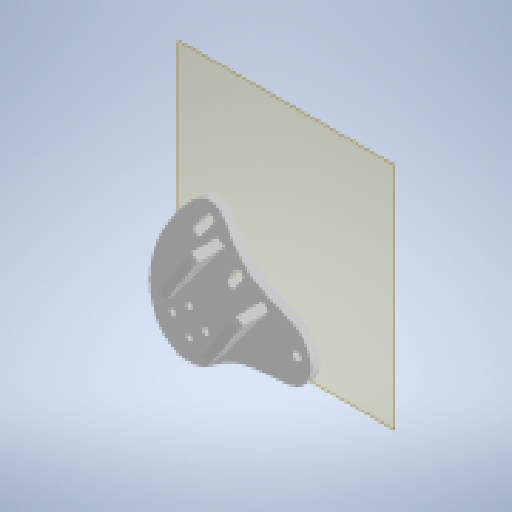
# Autodesk Inventor part: Soporte motor 2
Saved by Autodesk Inventor 2025.3 (Build 293356000, 356)
## iProperties
Created: 2025-11-13
Part Number: Soporte motor 2
Material: Generic
Document SubType Name: Modeling
Designer: juanm
Density: 1 g/cm^3
Appearance: Default
Author: juanm
Autodesk Inventor part; units mm, degrees
ref_plane "YZ Plane" through (0, 0, 0) normal (1, 0, 0) x (0, 1, 0)
ref_plane "XZ Plane" through (0, 0, 0) normal (0, 1, 0) x (-1, 0, 0)
ref_plane "XY Plane" through (0, 0, 0) normal (0, 0, 1) x (1, 0, 0)
ref_plane "Work Plane1" through (0, 0, 0) normal (0, 0, 1) x (1, 0, 0)
sketch "Sketch1" plane through (0, 0, 0) normal (0, 0, 1) x (1, 0, 0)
  circle A0 centre (-25.0838, -31.7051) radius 2.5 projected
  circle A1 centre (-43.012, -13.2629) radius 2.5 projected
  circle A2 centre (-44.8914, 13.7567) radius 2.5 projected
  circle A3 centre (-28.0838, 36.7109) radius 2.5 projected
  circle A4 centre (0.8935, 43.7288) radius 2.5 projected
  circle A5 centre (29.5533, 30.4373) radius 2.5 projected
  circle A6 centre (43.6662, -0.0951) radius 2.5 projected
  circle A7 centre (47.6662, -52.5951) radius 2.5 projected
  circle A8 centre (10.6662, -52.5951) radius 2.5 projected
  circle A9 centre (-6.8338, -0.0951) radius 8.75 projected
  line L0 (56.6662, -60.0951) -> (51.1662, -0.0951) projected
  spline S0 degree 4 poles (51.1662, -0.0951) (50.0319, 24.6801) (26.25, 55.8136) (-25.1104, 60.0951) (-56.6662, 18.5311) (-54.7055, -22.2338) (-29.645, -43.1708) (-8.3823, -44.3792) (3.1662, -40.8213) knots 0 0 0 0 0 0.330099 0.457579 0.582312 0.704438 0.895347 0.895347 0.895347 0.895347 0.895347 projected
  line L1 (3.1662, -40.8213) -> (3.1662, -60.0951) projected
  line L2 (3.1662, -60.0951) -> (56.6662, -60.0951) projected
  circle A10 centre (-6.8338, -0.0951) radius 80 construction
  circle A11 centre (-51.3856, -66.5416) radius 20
  spline S1 degree 4 poles (-67.6748, -78.146) (-80.1343, -60.6563) (-73.4442, -28.8039) (-34.6199, 23.5084) (-28.149, -22.306) (-1.1527, -34.0954) (21.6131, -40.077) (20.0804, -79.4594) (-16.1771, -65.3424) (-30.503, -75.865) (-39.3686, -82.5289) knots 0 0 0 0 0 0.227581 0.363335 0.480166 0.59047 0.703016 0.817261 1 1 1 1 1
  line L3 (10.6662, -52.5951) -> (-43.012, -13.2629) construction
  line L4 (-25.0838, -31.7051) -> (10.6662, -52.5951) construction
  line L5 (10.6662, -52.5951) -> (-42.0733, -6.3735) construction
  line L6 (10.6662, -52.5951) -> (-49.6403, -16.0265) construction
  arc A12 (-37.4996, -10.382) -> (-40.9954, -14.7405) centre (10.6662, -52.5951) ccw
  arc A13 (-40.9954, -14.7405) -> (-44.098, -19.3872) centre (10.6662, -52.5951) ccw
  arc A14 (-41.2598, -7.0865) -> (-45.0286, -11.7853) centre (10.6662, -52.5951) ccw
  arc A15 (-45.0286, -11.7853) -> (-48.3734, -16.7947) centre (10.6662, -52.5951) ccw
  arc A16 (-37.4996, -10.382) -> (-41.2598, -7.0865) centre (-39.3797, -8.7342) ccw
  arc A17 (-48.3734, -16.7947) -> (-44.098, -19.3872) centre (-46.2357, -18.0909) ccw
  line L7 (10.6662, -52.5951) -> (-30.2455, -33.2568) construction
  line L8 (10.6662, -52.5951) -> (-26.0132, -26.6253) construction
  arc A18 (-21.0867, -30.1134) -> (-24.5082, -35.9687) centre (10.6662, -52.5951) ccw
  arc A19 (-25.1674, -27.2241) -> (-29.0287, -33.832) centre (10.6662, -52.5951) ccw
  arc A20 (-21.0867, -30.1134) -> (-25.1674, -27.2241) centre (-23.1271, -28.6687) ccw
  arc A21 (-29.0287, -33.832) -> (-24.5082, -35.9687) centre (-26.7685, -34.9004) ccw
  point P0 (0, 0)
  point P1 (-60.5912, -17.8314)
  point P2 (-36.7792, -0.096)
  point P3 (-23.1279, -18.1974)
  point P4 (0.0342, -33.7731)
  point P5 (16.7837, -45.8922)
  point P6 (15.1081, -64.5601)
  point P7 (-10.6842, -70.5676)
  point P8 (-45.0286, -11.7853)
  point P9 (-21.0867, -30.1134)
  dimension "d0" = 160
  dimension "d1" = 40
  dimension "d2" = 5
  dimension "d3" = 5
  dimension "d4" = 2.5
  dimension "d5" = 5
  dimension "d6" = 5
  constraints: 27 point on circle, 15 point on line, 12 end point, 11 centre point, 7 coincident, 4 tangent, 13 other
  measures "d1" diameter of A11
  measures "d2" angle of L5 L3
  measures "d3" angle of L6 L3
  measures "d4" radius of A16
  measures "d5" angle of L4 L7
  measures "d6" angle of L4 L8
extrude "Extrusion1" add sketch "Sketch1" along normal blind 5 contours A15 A17 S0 S1 L2 L1 A13 A12 A16 A14 | A11 | A17 S0 L1 L2 S1 A11
sketch "Sketch2" plane through (0, 0, 0) normal (0, 0, -1) x (-1, 0, 0)
  arc A0 (39.3686, -82.5289) -> (67.6748, -78.146) centre (51.3856, -66.5416) ccw projected
  circle A1 centre (51.3856, -66.5416) radius 8 construction
  circle A2 centre (51.3856, -66.5416) radius 9.5 construction
  point P0 (0, 0)
  point P1 (60.8856, -66.5416)
  point P2 (41.8856, -66.5416)
  point P3 (51.3856, -74.5416)
  point P4 (51.3856, -58.5416)
  dimension "d9" = 16
  dimension "d10" = 19
  constraints: 4 point on circle, 2 centre point, 2 coincident
  measures "d9" diameter of A1
  measures "d10" diameter of A2
hole "Hole1" at (-60.8856, -66.5416, 0) at (-41.8856, -66.5416, 0) at (-51.3856, -74.5416, 0) at (-51.3856, -58.5416, 0) direction (0, 0, 1) diameter 3.7 end through all
sketch "Sketch3" plane through (0, 0, 0) normal (0, 0, -1) x (-1, 0, 0)
  circle A0 centre (51.3856, -58.5416) radius 1.85 projected
  circle A1 centre (51.3856, -74.5416) radius 1.85 projected
  circle A2 centre (41.8856, -66.5416) radius 1.85 projected
  circle A3 centre (60.8856, -66.5416) radius 1.85 projected
  arc A4 (39.3686, -82.5289) -> (67.6748, -78.146) centre (51.3856, -66.5416) ccw projected
  arc A5 (44.098, -19.3872) -> (48.3734, -16.7947) centre (46.2357, -18.0909) ccw projected
  arc A6 (44.098, -19.3872) -> (37.4996, -10.382) centre (-10.6662, -52.5951) ccw projected
  arc A7 (41.2598, -7.0865) -> (37.4996, -10.382) centre (39.3797, -8.7342) ccw projected
  arc A8 (48.3734, -16.7947) -> (41.2598, -7.0865) centre (-10.6662, -52.5951) ccw projected
  arc A9 (25.1674, -27.2241) -> (21.0867, -30.1134) centre (23.1271, -28.6687) ccw projected
  arc A10 (29.0287, -33.832) -> (25.1674, -27.2241) centre (-10.6662, -52.5951) ccw projected
  arc A11 (24.5082, -35.9687) -> (29.0287, -33.832) centre (26.7685, -34.9004) ccw projected
  arc A12 (24.5082, -35.9687) -> (21.0867, -30.1134) centre (-10.6662, -52.5951) ccw projected
  circle A13 centre (-10.6662, -52.5951) radius 2.5 projected
  circle A14 centre (60.8856, -66.5416) radius 4.5
  circle A15 centre (51.3856, -74.5416) radius 4.5
  circle A16 centre (41.8856, -66.5416) radius 4.5
  circle A17 centre (51.3856, -58.5416) radius 4.5
  point P0 (0, 0)
  dimension "d18" = 9
  dimension "d19" = 9
  dimension "d20" = 9
  dimension "d21" = 9
  constraints: 4 centre point, 4 coincident, 1 other
  measures "d18" diameter of A16
  measures "d19" diameter of A15
  measures "d20" diameter of A14
  measures "d21" diameter of A17
extrude "Extrusion2" add sketch "Sketch3" along normal blind 2 contours A14 | A15 | A16 | A17
sketch "Sketch4" plane through (0, 0, 5) normal (0, 0, 1) x (1, 0, 0)
  circle A0 centre (-51.3856, -58.5416) radius 1.85 projected
  circle A1 centre (-51.3856, -74.5416) radius 1.85 projected
  circle A2 centre (-41.8856, -66.5416) radius 1.85 projected
  circle A3 centre (-60.8856, -66.5416) radius 1.85 projected
  arc A4 (-67.6748, -78.146) -> (-39.3686, -82.5289) centre (-51.3856, -66.5416) ccw projected
  arc A5 (-48.3734, -16.7947) -> (-44.098, -19.3872) centre (-46.2357, -18.0909) ccw projected
  arc A6 (-41.2598, -7.0865) -> (-48.3734, -16.7947) centre (10.6662, -52.5951) ccw projected
  arc A7 (-37.4996, -10.382) -> (-41.2598, -7.0865) centre (-39.3797, -8.7342) ccw projected
  arc A8 (-37.4996, -10.382) -> (-44.098, -19.3872) centre (10.6662, -52.5951) ccw projected
  arc A9 (-21.0867, -30.1134) -> (-25.1674, -27.2241) centre (-23.1271, -28.6687) ccw projected
  arc A10 (-21.0867, -30.1134) -> (-24.5082, -35.9687) centre (10.6662, -52.5951) ccw projected
  arc A11 (-29.0287, -33.832) -> (-24.5082, -35.9687) centre (-26.7685, -34.9004) ccw projected
  arc A12 (-25.1674, -27.2241) -> (-29.0287, -33.832) centre (10.6662, -52.5951) ccw projected
  circle A13 centre (10.6662, -52.5951) radius 2.5 projected
  line L0 (-35.0492, -15.9402) -> (-63.5128, -53.8187)
  line L1 (-63.5128, -53.8187) -> (-59.5155, -56.8224)
  line L2 (-59.5155, -56.8224) -> (-31.0519, -18.9439)
  line L3 (-31.0519, -18.9439) -> (-35.0492, -15.9402)
  line L4 (-9.4669, -35.1638) -> (-38.9594, -74.4116)
  line L5 (-38.9594, -74.4116) -> (-34.9622, -77.4153)
  line L6 (-34.9622, -77.4153) -> (-5.4697, -38.1675)
  line L7 (-5.4697, -38.1675) -> (-9.4669, -35.1638)
  point P0 (0, 0)
  dimension "d24" = 5
  dimension "d25" = 5
  dimension "d26" = 27
  constraints: 16 end point, 6 perpendicular, 2 point on line, 1 other
  measures "d24" distance between parallel lines of L2 L0
  measures "d25" distance between parallel lines of L6 L4
  measures "d26" distance between parallel lines of L4 L2
extrude "Extrusion3" add sketch "Sketch4" along normal blind 15 contours L3 L2 L1 L0 | L7 L6 L5 L4
sketch "Sketch5" plane through (-63.5128, -53.8187, 5) normal (-0.7994, 0.6007, 0) x (0, 0, 1)
  line L0 (0, 0) -> (0, 47.381) projected
  line L1 (0, 0) -> (15, 0) projected
  line L2 (15, 47.381) -> (15, 0) projected
  line L3 (0, 47.381) -> (15, 47.381) projected
  line L4 (15, 0) -> (15, 47.381) projected
  line L5 (15, 42.381) -> (5, -1.85)
  line L6 (5, -1.85) -> (0, -1.85)
  line L7 (0, -1.85) -> (0, 0)
  line L8 (15, 42.381) -> (15, -1.85)
  line L9 (15, -1.85) -> (5, -1.85)
  point P0 (-5, 81.1797)
  dimension "d29" = 5
  dimension "d30" = 5
  constraints: 10 end point, 2 perpendicular, 2 point on line
  measures "d29" distance from line of L3 L5.start
  measures "d30" distance of L5.end L6.end
extrude "Extrusion4" cut sketch "Sketch5" against normal blind 41.9875 contours L5 L2 L1 | L1 L8 L9 L5
body "Solid1"
